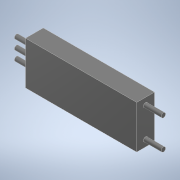
# Autodesk Inventor part: ESC
Saved by Autodesk Inventor 2022 (Build 260153000, 153)
## iProperties
Created: 2022-08-09
Part Number: ESC
Material: Generic
Document SubType Name: Modeling
Designer: Nick
Density: 1.62117 g/cm^3
Appearance: Smooth - Black
Mass: 43 g
Surface Area: 74.1149 cm^2
Volume: 26.5241 cm^3
Author: Nick
Autodesk Inventor part; units mm, degrees
ref_plane "YZ Plane" through (0, 0, 0) normal (1, 0, 0) x (0, 1, 0)
ref_plane "XZ Plane" through (0, 0, 0) normal (0, 1, 0) x (-1, 0, 0)
ref_plane "XY Plane" through (0, 0, 0) normal (0, 0, 1) x (1, 0, 0)
sketch "Sketch1" plane through (0, 0, 0) normal (0, 0, 1) x (1, 0, 0)
  line L0 (0, 0) -> (75, 0)
  line L1 (75, 0) -> (75, 29)
  line L2 (75, 29) -> (0, 29)
  line L3 (0, 29) -> (0, 0)
  dimension "d0" = 75
  dimension "d1" = 29
  constraints: 8 end point, 2 parallel, 1 horizontal, 1 perpendicular
  measures "d0" distance of L1.end L2.end
  measures "d1" distance of L0.end L1.end
extrude "Extrusion1" add sketch "Sketch1" along normal blind 12
sketch "Sketch2" plane through (75, 0, 0) normal (1, 0, 0) x (0, 0, -1)
  circle A0 centre (-6, 24.5) radius 1.5
  circle A1 centre (-6, 4.5) radius 1.5
  line L0 (0, 0) -> (-12, 0) projected
  line L1 (0, 29) -> (-12, 29) projected
  point P0 (-6, 0)
  dimension "d4" = 3
  dimension "d5" = 4.5
  dimension "d6" = 4.5
  constraints: 2 centre point, 2 vertical alignment, 1 equal radius, 1 midpoint
  measures "d4" diameter of A0
  measures "d5" distance from line of A0.centre L1
  measures "d6" distance from line of L0 A1.centre
extrude "Extrusion2" add sketch "Sketch2" along normal blind 12
sketch "Sketch3" plane through (0, 0, 0) normal (-1, 0, 0) x (0, 0, 1)
  circle A0 centre (6, 21) radius 1.5
  circle A1 centre (6, 14.5) radius 1.5
  circle A2 centre (6, 8) radius 1.5
  line L0 (0, 29) -> (12, 29) projected
  line L1 (6, 21) -> (6, 29) construction
  line L2 (6, 8) -> (6, 0) construction
  line L3 (0, 0) -> (12, 0) construction
  dimension "d9" = 6.5
  dimension "d10" = 6.5
  dimension "d11" = 3
  constraints: 4 end point, 3 centre point, 3 vertical alignment, 2 equal radius, 2 midpoint, 1 collinear, 1 vertical
  measures "d9" distance of L1.start A1.centre
  measures "d10" distance of L2.start A1.centre
  measures "d11" diameter of A0
extrude "Extrusion3" add sketch "Sketch3" along normal blind 12
equation "\"d6\" = d5"
equation "\"d10\" = d9"
body "Solid1"
